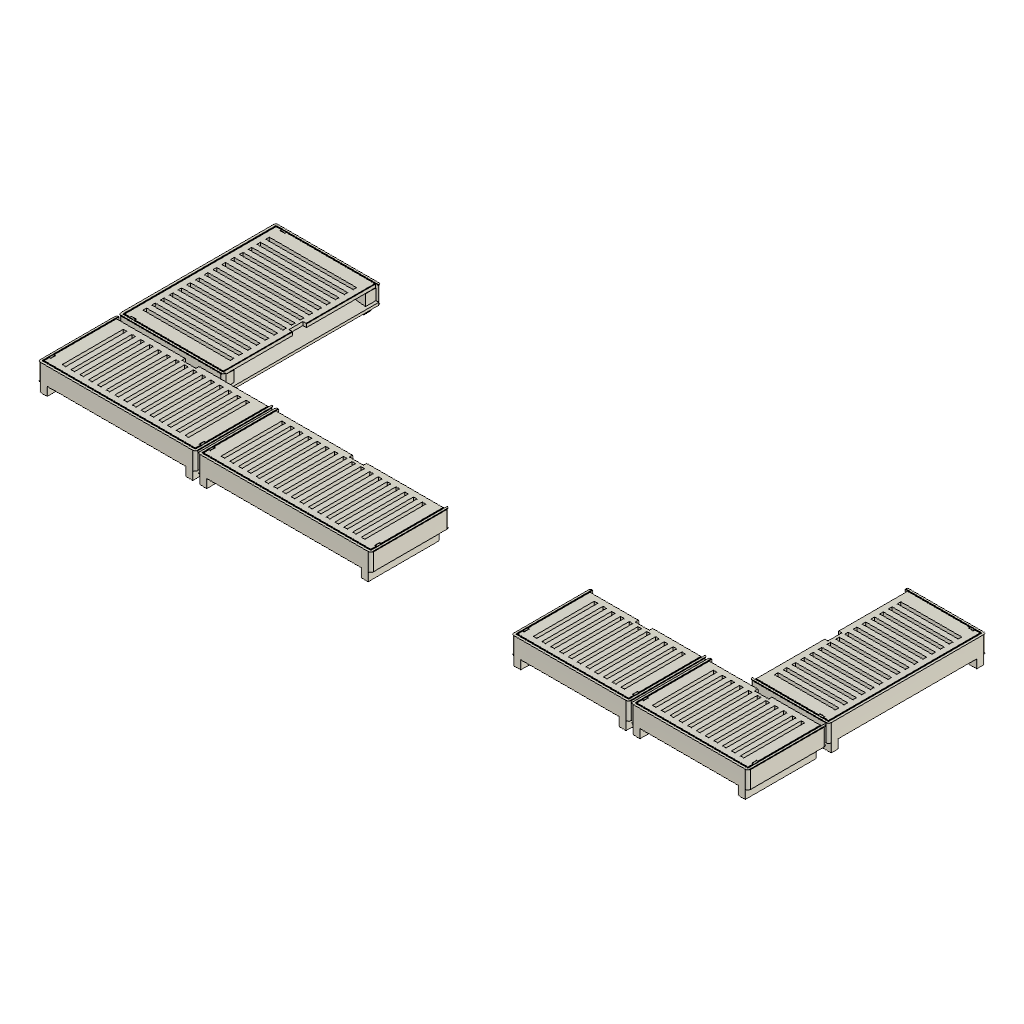
Sink_Organizer_B_R04_Single_Low (Autodesk Fusion 360 design; units mm, degrees)
Autodesk Fusion 360 part; units mm, degrees
(part 1 of 5)
ref_plane "工作平面1" through (0, 0, 10) normal (0, 0, 1) x (1, 0, 0) in component "R1_Integrated"
sketch "草图1" plane through (0, 0, 10) normal (0, 0, 1) x (1, 0, 0) in component "R1_Integrated"
  line L0 (590, 50) -> (724, 50)
  line L1 (724, 50) -> (724, 140)
  line L2 (724, 140) -> (590, 140)
  line L3 (590, 140) -> (590, 50)
  dimension "d43" = 590
  dimension "d44" = 50
  dimension "d45" = 134
  dimension "d46" = 90
  constraint horizontal L0
  constraint vertical L1
  constraint horizontal L2
  constraint vertical L3
  measures "d43" horizontal distance of origin L0.start
  measures "d44" vertical distance of origin L0.start
  measures "d45" horizontal distance of L0.start L0.end
  measures "d46" vertical distance of L0.end L1.end
extrude "R04 pan blank" add sketch "草图1" along normal blind 20 makes body 1 in component "R1_Integrated"
fillet "Outside corner rounds" radius 3 4 edges at (590, 140, 20) (724, 140, 20) (724, 50, 20) (590, 50, 20) on bodies 1 in component "R1_Integrated"
ref_plane "工作平面2" through (593, 0, 0) normal (1, 0, 0) x (0, 1, 0) in component "R1_Integrated"
sketch "草图2" plane through (593, 0, 0) normal (1, 0, 0) x (0, 0, -1) in component "R1_Integrated"
  line L0 (-22.1441, 53) -> (-13, 140)
  line L1 (-13, 140) -> (-31, 140)
  line L2 (-31, 140) -> (-31, 53)
  line L3 (-31, 53) -> (-22.1441, 53)
  dimension "d55" = 13
  dimension "d57" = 31
  constraint horizontal L1
  constraint vertical L2
  constraint horizontal L3
  measures "d55" horizontal distance of origin L0.end
  measures "d57" horizontal distance of origin L1.end
extrude "R04 continuous slope and open edge" cut sketch "草图2" along normal blind 128 bodies 1 in component "R1_Integrated"
ref_plane "工作平面3" through (0, 0, 10) normal (0, 0, 1) x (1, 0, 0) in component "R1_Integrated"
sketch "草图3" plane through (0, 0, 10) normal (0, 0, 1) x (1, 0, 0) in component "R1_Integrated"
  line L0 (593, 53) -> (605, 53)
  line L1 (605, 53) -> (605, 65)
  line L2 (605, 65) -> (593, 65)
  line L3 (593, 65) -> (593, 53)
  dimension "d64" = 12
  dimension "d65" = 12
  constraint horizontal L0
  constraint vertical L1
  constraint horizontal L2
  constraint vertical L3
  measures "d64" horizontal distance of L0.start L0.end
  measures "d65" vertical distance of L0.end L1.end
extrude "Grate seat 00" add sketch "草图3" along normal blind 16 bodies 1 in component "R1_Integrated"
ref_plane "工作平面4" through (0, 0, 10) normal (0, 0, 1) x (1, 0, 0) in component "R1_Integrated"
sketch "草图4" plane through (0, 0, 10) normal (0, 0, 1) x (1, 0, 0) in component "R1_Integrated"
  line L0 (593, 125) -> (605, 125)
  line L1 (605, 125) -> (605, 137)
  line L2 (605, 137) -> (593, 137)
  line L3 (593, 137) -> (593, 125)
  dimension "d71" = 125
  dimension "d72" = 12
  dimension "d73" = 12
  constraint horizontal L0
  constraint vertical L1
  constraint horizontal L2
  constraint vertical L3
  measures "d71" vertical distance of origin L0.start
  measures "d72" horizontal distance of L0.start L0.end
  measures "d73" vertical distance of L0.end L1.end
extrude "Grate seat 01" add sketch "草图4" along normal blind 16 bodies 1 in component "R1_Integrated"
ref_plane "工作平面5" through (0, 0, 10) normal (0, 0, 1) x (1, 0, 0) in component "R1_Integrated"
sketch "草图5" plane through (0, 0, 10) normal (0, 0, 1) x (1, 0, 0) in component "R1_Integrated"
  line L0 (709, 53) -> (721, 53)
  line L1 (721, 53) -> (721, 65)
  line L2 (721, 65) -> (709, 65)
  line L3 (709, 65) -> (709, 53)
  dimension "d78" = 709
  dimension "d80" = 12
  dimension "d81" = 12
  constraint horizontal L0
  constraint vertical L1
  constraint horizontal L2
  constraint vertical L3
  measures "d78" horizontal distance of origin L0.start
  measures "d80" horizontal distance of L0.start L0.end
  measures "d81" vertical distance of L0.end L1.end
extrude "Grate seat 10" add sketch "草图5" along normal blind 16 bodies 1 in component "R1_Integrated"
ref_plane "工作平面6" through (0, 0, 10) normal (0, 0, 1) x (1, 0, 0) in component "R1_Integrated"
sketch "草图6" plane through (0, 0, 10) normal (0, 0, 1) x (1, 0, 0) in component "R1_Integrated"
  line L0 (709, 125) -> (721, 125)
  line L1 (721, 125) -> (721, 137)
  line L2 (721, 137) -> (709, 137)
  line L3 (709, 137) -> (709, 125)
  dimension "d86" = 709
  dimension "d87" = 125
  dimension "d88" = 12
  dimension "d89" = 12
  constraint horizontal L0
  constraint vertical L1
  constraint horizontal L2
  constraint vertical L3
  measures "d86" horizontal distance of origin L0.start
  measures "d87" vertical distance of origin L0.start
  measures "d88" horizontal distance of L0.start L0.end
  measures "d89" vertical distance of L0.end L1.end
extrude "Grate seat 11" add sketch "草图6" along normal blind 16 bodies 1 in component "R1_Integrated"
ref_plane "工作平面7" through (0, 0, 0) normal (0, 0, 1) x (1, 0, 0) in component "R1_Integrated"
sketch "草图7" plane through (0, 0, 0) normal (0, 0, 1) x (1, 0, 0) in component "R1_Integrated"
  line L0 (593, 50) -> (601, 50)
  line L1 (601, 50) -> (601, 131)
  line L2 (601, 131) -> (593, 131)
  line L3 (593, 131) -> (593, 50)
  dimension "d94" = 593
  dimension "d95" = 50
  dimension "d96" = 8
  dimension "d97" = 81
  constraint horizontal L0
  constraint vertical L1
  constraint horizontal L2
  constraint vertical L3
  measures "d94" horizontal distance of origin L0.start
  measures "d95" vertical distance of origin L0.start
  measures "d96" horizontal distance of L0.start L0.end
  measures "d97" vertical distance of L0.end L1.end
extrude "R04 low integral runner 0" add sketch "草图7" along normal blind 10 bodies 1 in component "R1_Integrated"
ref_plane "工作平面8" through (0, 0, 0) normal (0, 0, 1) x (1, 0, 0) in component "R1_Integrated"
sketch "草图8" plane through (0, 0, 0) normal (0, 0, 1) x (1, 0, 0) in component "R1_Integrated"
  line L0 (713, 50) -> (721, 50)
  line L1 (721, 50) -> (721, 131)
  line L2 (721, 131) -> (713, 131)
  line L3 (713, 131) -> (713, 50)
  dimension "d102" = 713
  dimension "d103" = 50
  dimension "d104" = 8
  dimension "d105" = 81
  constraint horizontal L0
  constraint vertical L1
  constraint horizontal L2
  constraint vertical L3
  measures "d102" horizontal distance of origin L0.start
  measures "d103" vertical distance of origin L0.start
  measures "d104" horizontal distance of L0.start L0.end
  measures "d105" vertical distance of L0.end L1.end
extrude "R04 low integral runner 1" add sketch "草图8" along normal blind 10 bodies 1 in component "R1_Integrated"
chamfer "R03 touch edge chamfer" distance 0.4 angle 45 5 edges at (657, 53, 30) (593, 96.5, 30) (721, 96.5, 30) (590, 95, 30) (724, 95, 30) on bodies 1 in component "R1_Integrated"
ref_plane "工作平面1" through (0, 0, 26) normal (0, 0, 1) x (1, 0, 0) in component "R1_RemovableGrate"
sketch "草图1 (2)" plane through (0, 0, 26) normal (0, 0, 1) x (1, 0, 0) in component "R1_RemovableGrate"
  line L0 (593.3, 53.3) -> (720.7, 53.3)
  line L1 (720.7, 53.3) -> (720.7, 136.7)
  line L2 (720.7, 136.7) -> (593.3, 136.7)
  line L3 (593.3, 136.7) -> (593.3, 53.3)
  dimension "d113" = 127.4
  dimension "d114" = 83.4
  constraint horizontal L0
  constraint vertical L1
  constraint horizontal L2
  constraint vertical L3
  measures "d113" horizontal distance of L0.start L0.end
  measures "d114" vertical distance of L0.end L1.end
extrude "Horizontal removable deck" add sketch "草图1 (2)" along normal blind 4 separate body makes body 2 in component "R1_RemovableGrate"
ref_plane "工作平面2" through (0, 0, 26) normal (0, 0, 1) x (1, 0, 0) in component "R1_RemovableGrate"
sketch "草图2 (2)" plane through (0, 0, 26) normal (0, 0, 1) x (1, 0, 0) in component "R1_RemovableGrate"
  line L0 (605, 60.3) -> (609, 60.3)
  line L1 (609, 60.3) -> (609, 129.7)
  line L2 (609, 129.7) -> (605, 129.7)
  line L3 (605, 129.7) -> (605, 60.3)
  dimension "d119" = 605
  dimension "d121" = 4
  dimension "d122" = 69.4
  constraint horizontal L0
  constraint vertical L1
  constraint horizontal L2
  constraint vertical L3
  measures "d119" horizontal distance of origin L0.start
  measures "d121" horizontal distance of L0.start L0.end
  measures "d122" vertical distance of L0.end L1.end
extrude "Drain slot 1" cut sketch "草图2 (2)" along normal blind 4 bodies 2 in component "R1_RemovableGrate"
ref_plane "工作平面3" through (0, 0, 26) normal (0, 0, 1) x (1, 0, 0) in component "R1_RemovableGrate"
sketch "草图3 (2)" plane through (0, 0, 26) normal (0, 0, 1) x (1, 0, 0) in component "R1_RemovableGrate"
  line L0 (615, 60.3) -> (619, 60.3)
  line L1 (619, 60.3) -> (619, 129.7)
  line L2 (619, 129.7) -> (615, 129.7)
  line L3 (615, 129.7) -> (615, 60.3)
  dimension "d127" = 615
  dimension "d129" = 4
  dimension "d130" = 69.4
  constraint horizontal L0
  constraint vertical L1
  constraint horizontal L2
  constraint vertical L3
  measures "d127" horizontal distance of origin L0.start
  measures "d129" horizontal distance of L0.start L0.end
  measures "d130" vertical distance of L0.end L1.end
extrude "Drain slot 2" cut sketch "草图3 (2)" along normal blind 4 bodies 2 in component "R1_RemovableGrate"
ref_plane "工作平面4" through (0, 0, 26) normal (0, 0, 1) x (1, 0, 0) in component "R1_RemovableGrate"
sketch "草图4 (2)" plane through (0, 0, 26) normal (0, 0, 1) x (1, 0, 0) in component "R1_RemovableGrate"
  line L0 (625, 60.3) -> (629, 60.3)
  line L1 (629, 60.3) -> (629, 129.7)
  line L2 (629, 129.7) -> (625, 129.7)
  line L3 (625, 129.7) -> (625, 60.3)
  dimension "d135" = 625
  dimension "d137" = 4
  dimension "d138" = 69.4
  constraint horizontal L0
  constraint vertical L1
  constraint horizontal L2
  constraint vertical L3
  measures "d135" horizontal distance of origin L0.start
  measures "d137" horizontal distance of L0.start L0.end
  measures "d138" vertical distance of L0.end L1.end
extrude "Drain slot 3" cut sketch "草图4 (2)" along normal blind 4 bodies 2 in component "R1_RemovableGrate"
ref_plane "工作平面5" through (0, 0, 26) normal (0, 0, 1) x (1, 0, 0) in component "R1_RemovableGrate"
sketch "草图5 (2)" plane through (0, 0, 26) normal (0, 0, 1) x (1, 0, 0) in component "R1_RemovableGrate"
  line L0 (635, 60.3) -> (639, 60.3)
  line L1 (639, 60.3) -> (639, 129.7)
  line L2 (639, 129.7) -> (635, 129.7)
  line L3 (635, 129.7) -> (635, 60.3)
  dimension "d143" = 635
  dimension "d145" = 4
  dimension "d146" = 69.4
  constraint horizontal L0
  constraint vertical L1
  constraint horizontal L2
  constraint vertical L3
  measures "d143" horizontal distance of origin L0.start
  measures "d145" horizontal distance of L0.start L0.end
  measures "d146" vertical distance of L0.end L1.end
extrude "Drain slot 4" cut sketch "草图5 (2)" along normal blind 4 bodies 2 in component "R1_RemovableGrate"
ref_plane "工作平面6" through (0, 0, 26) normal (0, 0, 1) x (1, 0, 0) in component "R1_RemovableGrate"
sketch "草图6 (2)" plane through (0, 0, 26) normal (0, 0, 1) x (1, 0, 0) in component "R1_RemovableGrate"
  line L0 (645, 60.3) -> (649, 60.3)
  line L1 (649, 60.3) -> (649, 129.7)
  line L2 (649, 129.7) -> (645, 129.7)
  line L3 (645, 129.7) -> (645, 60.3)
  dimension "d151" = 645
  dimension "d153" = 4
  dimension "d154" = 69.4
  constraint horizontal L0
  constraint vertical L1
  constraint horizontal L2
  constraint vertical L3
  measures "d151" horizontal distance of origin L0.start
  measures "d153" horizontal distance of L0.start L0.end
  measures "d154" vertical distance of L0.end L1.end
extrude "Drain slot 5" cut sketch "草图6 (2)" along normal blind 4 bodies 2 in component "R1_RemovableGrate"
ref_plane "工作平面7" through (0, 0, 26) normal (0, 0, 1) x (1, 0, 0) in component "R1_RemovableGrate"
sketch "草图7 (2)" plane through (0, 0, 26) normal (0, 0, 1) x (1, 0, 0) in component "R1_RemovableGrate"
  line L0 (655, 60.3) -> (659, 60.3)
  line L1 (659, 60.3) -> (659, 129.7)
  line L2 (659, 129.7) -> (655, 129.7)
  line L3 (655, 129.7) -> (655, 60.3)
  dimension "d159" = 655
  dimension "d161" = 4
  dimension "d162" = 69.4
  constraint horizontal L0
  constraint vertical L1
  constraint horizontal L2
  constraint vertical L3
  measures "d159" horizontal distance of origin L0.start
  measures "d161" horizontal distance of L0.start L0.end
  measures "d162" vertical distance of L0.end L1.end
extrude "Drain slot 6" cut sketch "草图7 (2)" along normal blind 4 bodies 2 in component "R1_RemovableGrate"
ref_plane "工作平面8" through (0, 0, 26) normal (0, 0, 1) x (1, 0, 0) in component "R1_RemovableGrate"
sketch "草图8 (2)" plane through (0, 0, 26) normal (0, 0, 1) x (1, 0, 0) in component "R1_RemovableGrate"
  line L0 (665, 60.3) -> (669, 60.3)
  line L1 (669, 60.3) -> (669, 129.7)
  line L2 (669, 129.7) -> (665, 129.7)
  line L3 (665, 129.7) -> (665, 60.3)
  dimension "d167" = 665
  dimension "d169" = 4
  dimension "d170" = 69.4
  constraint horizontal L0
  constraint vertical L1
  constraint horizontal L2
  constraint vertical L3
  measures "d167" horizontal distance of origin L0.start
  measures "d169" horizontal distance of L0.start L0.end
  measures "d170" vertical distance of L0.end L1.end
extrude "Drain slot 7" cut sketch "草图8 (2)" along normal blind 4 bodies 2 in component "R1_RemovableGrate"
ref_plane "工作平面9" through (0, 0, 26) normal (0, 0, 1) x (1, 0, 0) in component "R1_RemovableGrate"
sketch "草图9" plane through (0, 0, 26) normal (0, 0, 1) x (1, 0, 0) in component "R1_RemovableGrate"
  line L0 (675, 60.3) -> (679, 60.3)
  line L1 (679, 60.3) -> (679, 129.7)
  line L2 (679, 129.7) -> (675, 129.7)
  line L3 (675, 129.7) -> (675, 60.3)
  dimension "d175" = 675
  dimension "d177" = 4
  dimension "d178" = 69.4
  constraint horizontal L0
  constraint vertical L1
  constraint horizontal L2
  constraint vertical L3
  measures "d175" horizontal distance of origin L0.start
  measures "d177" horizontal distance of L0.start L0.end
  measures "d178" vertical distance of L0.end L1.end
extrude "Drain slot 8" cut sketch "草图9" along normal blind 4 bodies 2 in component "R1_RemovableGrate"
ref_plane "工作平面10" through (0, 0, 26) normal (0, 0, 1) x (1, 0, 0) in component "R1_RemovableGrate"
sketch "草图10" plane through (0, 0, 26) normal (0, 0, 1) x (1, 0, 0) in component "R1_RemovableGrate"
  line L0 (685, 60.3) -> (689, 60.3)
  line L1 (689, 60.3) -> (689, 129.7)
  line L2 (689, 129.7) -> (685, 129.7)
  line L3 (685, 129.7) -> (685, 60.3)
  dimension "d183" = 685
  dimension "d185" = 4
  dimension "d186" = 69.4
  constraint horizontal L0
  constraint vertical L1
  constraint horizontal L2
  constraint vertical L3
  measures "d183" horizontal distance of origin L0.start
  measures "d185" horizontal distance of L0.start L0.end
  measures "d186" vertical distance of L0.end L1.end
extrude "Drain slot 9" cut sketch "草图10" along normal blind 4 bodies 2 in component "R1_RemovableGrate"
ref_plane "工作平面11" through (0, 0, 26) normal (0, 0, 1) x (1, 0, 0) in component "R1_RemovableGrate"
sketch "草图11" plane through (0, 0, 26) normal (0, 0, 1) x (1, 0, 0) in component "R1_RemovableGrate"
  line L0 (695, 60.3) -> (699, 60.3)
  line L1 (699, 60.3) -> (699, 129.7)
  line L2 (699, 129.7) -> (695, 129.7)
  line L3 (695, 129.7) -> (695, 60.3)
  dimension "d191" = 695
  dimension "d193" = 4
  dimension "d194" = 69.4
  constraint horizontal L0
  constraint vertical L1
  constraint horizontal L2
  constraint vertical L3
  measures "d191" horizontal distance of origin L0.start
  measures "d193" horizontal distance of L0.start L0.end
  measures "d194" vertical distance of L0.end L1.end
extrude "Drain slot 10" cut sketch "草图11" along normal blind 4 bodies 2 in component "R1_RemovableGrate"
ref_plane "工作平面12" through (0, 0, 26) normal (0, 0, 1) x (1, 0, 0) in component "R1_RemovableGrate"
sketch "草图12" plane through (0, 0, 26) normal (0, 0, 1) x (1, 0, 0) in component "R1_RemovableGrate"
  line L0 (705, 60.3) -> (709, 60.3)
  line L1 (709, 60.3) -> (709, 129.7)
  line L2 (709, 129.7) -> (705, 129.7)
  line L3 (705, 129.7) -> (705, 60.3)
  dimension "d199" = 705
  dimension "d201" = 4
  dimension "d202" = 69.4
  constraint horizontal L0
  constraint vertical L1
  constraint horizontal L2
  constraint vertical L3
  measures "d199" horizontal distance of origin L0.start
  measures "d201" horizontal distance of L0.start L0.end
  measures "d202" vertical distance of L0.end L1.end
extrude "Drain slot 11" cut sketch "草图12" along normal blind 4 bodies 2 in component "R1_RemovableGrate"
ref_plane "工作平面13" through (0, 0, 26) normal (0, 0, 1) x (1, 0, 0) in component "R1_RemovableGrate"
sketch "草图13" plane through (0, 0, 26) normal (0, 0, 1) x (1, 0, 0) in component "R1_RemovableGrate"
  line L0 (649, 132.7) -> (665, 132.7)
  line L1 (665, 132.7) -> (665, 137.7)
  line L2 (665, 137.7) -> (649, 137.7)
  line L3 (649, 137.7) -> (649, 132.7)
  dimension "d207" = 649
  dimension "d208" = 132.7
  dimension "d209" = 16
  dimension "d210" = 5
  constraint horizontal L0
  constraint vertical L1
  constraint horizontal L2
  constraint vertical L3
  measures "d207" horizontal distance of origin L0.start
  measures "d208" vertical distance of origin L0.start
  measures "d209" horizontal distance of L0.start L0.end
  measures "d210" vertical distance of L0.end L1.end
extrude "Finger lift notch" cut sketch "草图13" along normal blind 4 bodies 2 in component "R1_RemovableGrate"
chamfer "R03 touch edge chamfer'" distance 0.4 angle 45 5 edges at (621.15, 136.7, 30) (593.3, 95, 30) (657, 53.3, 30) (720.7, 95, 30) (692.85, 136.7, 30) on bodies 2 in component "R1_RemovableGrate"
ref_plane "工作平面1" through (0, 0, 10) normal (0, 0, 1) x (1, 0, 0) in component "L1_Integrated"
sketch "草图1 (3)" plane through (0, 0, 10) normal (0, 0, 1) x (1, 0, 0) in component "L1_Integrated"
  line L0 (50, 50) -> (230, 50)
  line L1 (230, 50) -> (230, 140)
  line L2 (230, 140) -> (50, 140)
  line L3 (50, 140) -> (50, 50)
  dimension "d216" = 50
  dimension "d217" = 50
  dimension "d218" = 180
  dimension "d219" = 90
  constraint horizontal L0
  constraint vertical L1
  constraint horizontal L2
  constraint vertical L3
  measures "d216" horizontal distance of origin L0.start
  measures "d217" vertical distance of origin L0.start
  measures "d218" horizontal distance of L0.start L0.end
  measures "d219" vertical distance of L0.end L1.end
extrude "R04 pan blank'" add sketch "草图1 (3)" along normal blind 20 separate body makes body 3 in component "L1_Integrated"
fillet "Outside corner rounds'" radius 3 4 edges at (50, 140, 20) (230, 140, 20) (230, 50, 20) (50, 50, 20) on bodies 3 in component "L1_Integrated"
ref_plane "工作平面2" through (53, 0, 0) normal (1, 0, 0) x (0, 1, 0) in component "L1_Integrated"
sketch "草图2 (3)" plane through (53, 0, 0) normal (1, 0, 0) x (0, 0, -1) in component "L1_Integrated"
  line L0 (-22.1441, 53) -> (-13, 140)
  line L1 (-13, 140) -> (-31, 140)
  line L2 (-31, 140) -> (-31, 53)
  line L3 (-31, 53) -> (-22.1441, 53)
  dimension "d228" = 13
  dimension "d230" = 31
  constraint horizontal L1
  constraint vertical L2
  constraint horizontal L3
  measures "d228" horizontal distance of origin L0.end
  measures "d230" horizontal distance of origin L1.end
extrude "R04 continuous slope and open edge'" cut sketch "草图2 (3)" along normal blind 174 bodies 3 in component "L1_Integrated"
ref_plane "工作平面3" through (0, 0, 10) normal (0, 0, 1) x (1, 0, 0) in component "L1_Integrated"
sketch "草图3 (3)" plane through (0, 0, 10) normal (0, 0, 1) x (1, 0, 0) in component "L1_Integrated"
  line L0 (53, 53) -> (65, 53)
  line L1 (65, 53) -> (65, 65)
  line L2 (65, 65) -> (53, 65)
  line L3 (53, 65) -> (53, 53)
  dimension "d237" = 12
  dimension "d238" = 12
  constraint horizontal L0
  constraint vertical L1
  constraint horizontal L2
  constraint vertical L3
  measures "d237" horizontal distance of L0.start L0.end
  measures "d238" vertical distance of L0.end L1.end
extrude "Grate seat 00'" add sketch "草图3 (3)" along normal blind 16 bodies 3 in component "L1_Integrated"
ref_plane "工作平面4" through (0, 0, 10) normal (0, 0, 1) x (1, 0, 0) in component "L1_Integrated"
sketch "草图4 (3)" plane through (0, 0, 10) normal (0, 0, 1) x (1, 0, 0) in component "L1_Integrated"
  line L0 (53, 125) -> (65, 125)
  line L1 (65, 125) -> (65, 137)
  line L2 (65, 137) -> (53, 137)
  line L3 (53, 137) -> (53, 125)
  dimension "d244" = 125
  dimension "d245" = 12
  dimension "d246" = 12
  constraint horizontal L0
  constraint vertical L1
  constraint horizontal L2
  constraint vertical L3
  measures "d244" vertical distance of origin L0.start
  measures "d245" horizontal distance of L0.start L0.end
  measures "d246" vertical distance of L0.end L1.end
extrude "Grate seat 01'" add sketch "草图4 (3)" along normal blind 16 bodies 3 in component "L1_Integrated"
ref_plane "工作平面5" through (0, 0, 10) normal (0, 0, 1) x (1, 0, 0) in component "L1_Integrated"
sketch "草图5 (3)" plane through (0, 0, 10) normal (0, 0, 1) x (1, 0, 0) in component "L1_Integrated"
  line L0 (215, 53) -> (227, 53)
  line L1 (227, 53) -> (227, 65)
  line L2 (227, 65) -> (215, 65)
  line L3 (215, 65) -> (215, 53)
  dimension "d251" = 215
  dimension "d253" = 12
  dimension "d254" = 12
  constraint horizontal L0
  constraint vertical L1
  constraint horizontal L2
  constraint vertical L3
  measures "d251" horizontal distance of origin L0.start
  measures "d253" horizontal distance of L0.start L0.end
  measures "d254" vertical distance of L0.end L1.end
extrude "Grate seat 10'" add sketch "草图5 (3)" along normal blind 16 bodies 3 in component "L1_Integrated"
ref_plane "工作平面6" through (0, 0, 10) normal (0, 0, 1) x (1, 0, 0) in component "L1_Integrated"
sketch "草图6 (3)" plane through (0, 0, 10) normal (0, 0, 1) x (1, 0, 0) in component "L1_Integrated"
  line L0 (215, 125) -> (227, 125)
  line L1 (227, 125) -> (227, 137)
  line L2 (227, 137) -> (215, 137)
  line L3 (215, 137) -> (215, 125)
  dimension "d259" = 215
  dimension "d260" = 125
  dimension "d261" = 12
  dimension "d262" = 12
  constraint horizontal L0
  constraint vertical L1
  constraint horizontal L2
  constraint vertical L3
  measures "d259" horizontal distance of origin L0.start
  measures "d260" vertical distance of origin L0.start
  measures "d261" horizontal distance of L0.start L0.end
  measures "d262" vertical distance of L0.end L1.end
extrude "Grate seat 11'" add sketch "草图6 (3)" along normal blind 16 bodies 3 in component "L1_Integrated"
ref_plane "工作平面7" through (0, 0, 0) normal (0, 0, 1) x (1, 0, 0) in component "L1_Integrated"
sketch "草图7 (3)" plane through (0, 0, 0) normal (0, 0, 1) x (1, 0, 0) in component "L1_Integrated"
  line L0 (53, 50) -> (61, 50)
  line L1 (61, 50) -> (61, 131)
  line L2 (61, 131) -> (53, 131)
  line L3 (53, 131) -> (53, 50)
  dimension "d267" = 53
  dimension "d268" = 50
  dimension "d269" = 8
  dimension "d270" = 81
  constraint horizontal L0
  constraint vertical L1
  constraint horizontal L2
  constraint vertical L3
  measures "d267" horizontal distance of origin L0.start
  measures "d268" vertical distance of origin L0.start
  measures "d269" horizontal distance of L0.start L0.end
  measures "d270" vertical distance of L0.end L1.end
extrude "R04 low integral runner 0'" add sketch "草图7 (3)" along normal blind 10 bodies 3 in component "L1_Integrated"
ref_plane "工作平面8" through (0, 0, 0) normal (0, 0, 1) x (1, 0, 0) in component "L1_Integrated"
sketch "草图8 (3)" plane through (0, 0, 0) normal (0, 0, 1) x (1, 0, 0) in component "L1_Integrated"
  line L0 (219, 50) -> (227, 50)
  line L1 (227, 50) -> (227, 131)
  line L2 (227, 131) -> (219, 131)
  line L3 (219, 131) -> (219, 50)
  dimension "d275" = 219
  dimension "d276" = 50
  dimension "d277" = 8
  dimension "d278" = 81
  constraint horizontal L0
  constraint vertical L1
  constraint horizontal L2
  constraint vertical L3
  measures "d275" horizontal distance of origin L0.start
  measures "d276" vertical distance of origin L0.start
  measures "d277" horizontal distance of L0.start L0.end
  measures "d278" vertical distance of L0.end L1.end
extrude "R04 low integral runner 1'" add sketch "草图8 (3)" along normal blind 10 bodies 3 in component "L1_Integrated"
chamfer "R03 touch edge chamfer''" distance 0.4 angle 45 5 edges at (140, 53, 30) (53, 96.5, 30) (227, 96.5, 30) (50, 95, 30) (230, 95, 30) on bodies 3 in component "L1_Integrated"
ref_plane "工作平面1" through (0, 0, 26) normal (0, 0, 1) x (1, 0, 0) in component "L1_RemovableGrate"
sketch "草图1 (4)" plane through (0, 0, 26) normal (0, 0, 1) x (1, 0, 0) in component "L1_RemovableGrate"
  line L0 (53.3, 53.3) -> (226.7, 53.3)
  line L1 (226.7, 53.3) -> (226.7, 136.7)
  line L2 (226.7, 136.7) -> (53.3, 136.7)
  line L3 (53.3, 136.7) -> (53.3, 53.3)
  dimension "d286" = 173.4
  dimension "d287" = 83.4
  constraint horizontal L0
  constraint vertical L1
  constraint horizontal L2
  constraint vertical L3
  measures "d286" horizontal distance of L0.start L0.end
  measures "d287" vertical distance of L0.end L1.end
extrude "Horizontal removable deck'" add sketch "草图1 (4)" along normal blind 4 separate body makes body 4 in component "L1_RemovableGrate"
ref_plane "工作平面2" through (0, 0, 26) normal (0, 0, 1) x (1, 0, 0) in component "L1_RemovableGrate"
sketch "草图2 (4)" plane through (0, 0, 26) normal (0, 0, 1) x (1, 0, 0) in component "L1_RemovableGrate"
  line L0 (68, 60.3) -> (72, 60.3)
  line L1 (72, 60.3) -> (72, 129.7)
  line L2 (72, 129.7) -> (68, 129.7)
  line L3 (68, 129.7) -> (68, 60.3)
  dimension "d292" = 68
  dimension "d294" = 4
  dimension "d295" = 69.4
  constraint horizontal L0
  constraint vertical L1
  constraint horizontal L2
  constraint vertical L3
  measures "d292" horizontal distance of origin L0.start
  measures "d294" horizontal distance of L0.start L0.end
  measures "d295" vertical distance of L0.end L1.end
extrude "Drain slot 1'" cut sketch "草图2 (4)" along normal blind 4 bodies 4 in component "L1_RemovableGrate"
ref_plane "工作平面3" through (0, 0, 26) normal (0, 0, 1) x (1, 0, 0) in component "L1_RemovableGrate"
sketch "草图3 (4)" plane through (0, 0, 26) normal (0, 0, 1) x (1, 0, 0) in component "L1_RemovableGrate"
  line L0 (78, 60.3) -> (82, 60.3)
  line L1 (82, 60.3) -> (82, 129.7)
  line L2 (82, 129.7) -> (78, 129.7)
  line L3 (78, 129.7) -> (78, 60.3)
  dimension "d300" = 78
  dimension "d302" = 4
  dimension "d303" = 69.4
  constraint horizontal L0
  constraint vertical L1
  constraint horizontal L2
  constraint vertical L3
  measures "d300" horizontal distance of origin L0.start
  measures "d302" horizontal distance of L0.start L0.end
  measures "d303" vertical distance of L0.end L1.end
extrude "Drain slot 2'" cut sketch "草图3 (4)" along normal blind 4 bodies 4 in component "L1_RemovableGrate"
ref_plane "工作平面4" through (0, 0, 26) normal (0, 0, 1) x (1, 0, 0) in component "L1_RemovableGrate"
sketch "草图4 (4)" plane through (0, 0, 26) normal (0, 0, 1) x (1, 0, 0) in component "L1_RemovableGrate"
  line L0 (88, 60.3) -> (92, 60.3)
  line L1 (92, 60.3) -> (92, 129.7)
  line L2 (92, 129.7) -> (88, 129.7)
  line L3 (88, 129.7) -> (88, 60.3)
  dimension "d308" = 88
  dimension "d310" = 4
  dimension "d311" = 69.4
  constraint horizontal L0
  constraint vertical L1
  constraint horizontal L2
  constraint vertical L3
  measures "d308" horizontal distance of origin L0.start
  measures "d310" horizontal distance of L0.start L0.end
  measures "d311" vertical distance of L0.end L1.end
extrude "Drain slot 3'" cut sketch "草图4 (4)" along normal blind 4 bodies 4 in component "L1_RemovableGrate"
ref_plane "工作平面5" through (0, 0, 26) normal (0, 0, 1) x (1, 0, 0) in component "L1_RemovableGrate"
sketch "草图5 (4)" plane through (0, 0, 26) normal (0, 0, 1) x (1, 0, 0) in component "L1_RemovableGrate"
  line L0 (98, 60.3) -> (102, 60.3)
  line L1 (102, 60.3) -> (102, 129.7)
  line L2 (102, 129.7) -> (98, 129.7)
  line L3 (98, 129.7) -> (98, 60.3)
  dimension "d316" = 98
  dimension "d318" = 4
  dimension "d319" = 69.4
  constraint horizontal L0
  constraint vertical L1
  constraint horizontal L2
  constraint vertical L3
  measures "d316" horizontal distance of origin L0.start
  measures "d318" horizontal distance of L0.start L0.end
  measures "d319" vertical distance of L0.end L1.end
extrude "Drain slot 4'" cut sketch "草图5 (4)" along normal blind 4 bodies 4 in component "L1_RemovableGrate"
ref_plane "工作平面6" through (0, 0, 26) normal (0, 0, 1) x (1, 0, 0) in component "L1_RemovableGrate"
sketch "草图6 (4)" plane through (0, 0, 26) normal (0, 0, 1) x (1, 0, 0) in component "L1_RemovableGrate"
  line L0 (108, 60.3) -> (112, 60.3)
  line L1 (112, 60.3) -> (112, 129.7)
  line L2 (112, 129.7) -> (108, 129.7)
  line L3 (108, 129.7) -> (108, 60.3)
  dimension "d324" = 108
  dimension "d326" = 4
  dimension "d327" = 69.4
  constraint horizontal L0
  constraint vertical L1
  constraint horizontal L2
  constraint vertical L3
  measures "d324" horizontal distance of origin L0.start
  measures "d326" horizontal distance of L0.start L0.end
  measures "d327" vertical distance of L0.end L1.end
extrude "Drain slot 5'" cut sketch "草图6 (4)" along normal blind 4 bodies 4 in component "L1_RemovableGrate"
ref_plane "工作平面7" through (0, 0, 26) normal (0, 0, 1) x (1, 0, 0) in component "L1_RemovableGrate"
sketch "草图7 (4)" plane through (0, 0, 26) normal (0, 0, 1) x (1, 0, 0) in component "L1_RemovableGrate"
  line L0 (118, 60.3) -> (122, 60.3)
  line L1 (122, 60.3) -> (122, 129.7)
  line L2 (122, 129.7) -> (118, 129.7)
  line L3 (118, 129.7) -> (118, 60.3)
  dimension "d332" = 118
  dimension "d334" = 4
  dimension "d335" = 69.4
  constraint horizontal L0
  constraint vertical L1
  constraint horizontal L2
  constraint vertical L3
  measures "d332" horizontal distance of origin L0.start
  measures "d334" horizontal distance of L0.start L0.end
  measures "d335" vertical distance of L0.end L1.end
extrude "Drain slot 6'" cut sketch "草图7 (4)" along normal blind 4 bodies 4 in component "L1_RemovableGrate"
ref_plane "工作平面8" through (0, 0, 26) normal (0, 0, 1) x (1, 0, 0) in component "L1_RemovableGrate"
sketch "草图8 (4)" plane through (0, 0, 26) normal (0, 0, 1) x (1, 0, 0) in component "L1_RemovableGrate"
  line L0 (128, 60.3) -> (132, 60.3)
  line L1 (132, 60.3) -> (132, 129.7)
  line L2 (132, 129.7) -> (128, 129.7)
  line L3 (128, 129.7) -> (128, 60.3)
  dimension "d340" = 128
  dimension "d342" = 4
  dimension "d343" = 69.4
  constraint horizontal L0
  constraint vertical L1
  constraint horizontal L2
  constraint vertical L3
  measures "d340" horizontal distance of origin L0.start
  measures "d342" horizontal distance of L0.start L0.end
  measures "d343" vertical distance of L0.end L1.end
extrude "Drain slot 7'" cut sketch "草图8 (4)" along normal blind 4 bodies 4 in component "L1_RemovableGrate"
ref_plane "工作平面9" through (0, 0, 26) normal (0, 0, 1) x (1, 0, 0) in component "L1_RemovableGrate"
sketch "草图9 (2)" plane through (0, 0, 26) normal (0, 0, 1) x (1, 0, 0) in component "L1_RemovableGrate"
  line L0 (138, 60.3) -> (142, 60.3)
  line L1 (142, 60.3) -> (142, 129.7)
  line L2 (142, 129.7) -> (138, 129.7)
  line L3 (138, 129.7) -> (138, 60.3)
  dimension "d348" = 138
  dimension "d350" = 4
  dimension "d351" = 69.4
  constraint horizontal L0
  constraint vertical L1
  constraint horizontal L2
  constraint vertical L3
  measures "d348" horizontal distance of origin L0.start
  measures "d350" horizontal distance of L0.start L0.end
  measures "d351" vertical distance of L0.end L1.end
extrude "Drain slot 8'" cut sketch "草图9 (2)" along normal blind 4 bodies 4 in component "L1_RemovableGrate"
ref_plane "工作平面10" through (0, 0, 26) normal (0, 0, 1) x (1, 0, 0) in component "L1_RemovableGrate"
sketch "草图10 (2)" plane through (0, 0, 26) normal (0, 0, 1) x (1, 0, 0) in component "L1_RemovableGrate"
  line L0 (148, 60.3) -> (152, 60.3)
  line L1 (152, 60.3) -> (152, 129.7)
  line L2 (152, 129.7) -> (148, 129.7)
  line L3 (148, 129.7) -> (148, 60.3)
  dimension "d356" = 148
  dimension "d358" = 4
  dimension "d359" = 69.4
  constraint horizontal L0
  constraint vertical L1
  constraint horizontal L2
  constraint vertical L3
  measures "d356" horizontal distance of origin L0.start
  measures "d358" horizontal distance of L0.start L0.end
  measures "d359" vertical distance of L0.end L1.end
extrude "Drain slot 9'" cut sketch "草图10 (2)" along normal blind 4 bodies 4 in component "L1_RemovableGrate"
ref_plane "工作平面11" through (0, 0, 26) normal (0, 0, 1) x (1, 0, 0) in component "L1_RemovableGrate"
sketch "草图11 (2)" plane through (0, 0, 26) normal (0, 0, 1) x (1, 0, 0) in component "L1_RemovableGrate"
  line L0 (158, 60.3) -> (162, 60.3)
  line L1 (162, 60.3) -> (162, 129.7)
  line L2 (162, 129.7) -> (158, 129.7)
  line L3 (158, 129.7) -> (158, 60.3)
  dimension "d364" = 158
  dimension "d366" = 4
  dimension "d367" = 69.4
  constraint horizontal L0
  constraint vertical L1
  constraint horizontal L2
  constraint vertical L3
  measures "d364" horizontal distance of origin L0.start
  measures "d366" horizontal distance of L0.start L0.end
  measures "d367" vertical distance of L0.end L1.end
extrude "Drain slot 10'" cut sketch "草图11 (2)" along normal blind 4 bodies 4 in component "L1_RemovableGrate"
ref_plane "工作平面12" through (0, 0, 26) normal (0, 0, 1) x (1, 0, 0) in component "L1_RemovableGrate"
sketch "草图12 (2)" plane through (0, 0, 26) normal (0, 0, 1) x (1, 0, 0) in component "L1_RemovableGrate"
  line L0 (168, 60.3) -> (172, 60.3)
  line L1 (172, 60.3) -> (172, 129.7)
  line L2 (172, 129.7) -> (168, 129.7)
  line L3 (168, 129.7) -> (168, 60.3)
  dimension "d372" = 168
  dimension "d374" = 4
  dimension "d375" = 69.4
  constraint horizontal L0
  constraint vertical L1
  constraint horizontal L2
  constraint vertical L3
  measures "d372" horizontal distance of origin L0.start
  measures "d374" horizontal distance of L0.start L0.end
  measures "d375" vertical distance of L0.end L1.end
extrude "Drain slot 11'" cut sketch "草图12 (2)" along normal blind 4 bodies 4 in component "L1_RemovableGrate"
ref_plane "工作平面13" through (0, 0, 26) normal (0, 0, 1) x (1, 0, 0) in component "L1_RemovableGrate"
sketch "草图13 (2)" plane through (0, 0, 26) normal (0, 0, 1) x (1, 0, 0) in component "L1_RemovableGrate"
  line L0 (178, 60.3) -> (182, 60.3)
  line L1 (182, 60.3) -> (182, 129.7)
  line L2 (182, 129.7) -> (178, 129.7)
  line L3 (178, 129.7) -> (178, 60.3)
  dimension "d380" = 178
  dimension "d382" = 4
  dimension "d383" = 69.4
  constraint horizontal L0
  constraint vertical L1
  constraint horizontal L2
  constraint vertical L3
  measures "d380" horizontal distance of origin L0.start
  measures "d382" horizontal distance of L0.start L0.end
  measures "d383" vertical distance of L0.end L1.end
extrude "Drain slot 12" cut sketch "草图13 (2)" along normal blind 4 bodies 4 in component "L1_RemovableGrate"
ref_plane "工作平面14" through (0, 0, 26) normal (0, 0, 1) x (1, 0, 0) in component "L1_RemovableGrate"
sketch "草图14" plane through (0, 0, 26) normal (0, 0, 1) x (1, 0, 0) in component "L1_RemovableGrate"
  line L0 (188, 60.3) -> (192, 60.3)
  line L1 (192, 60.3) -> (192, 129.7)
  line L2 (192, 129.7) -> (188, 129.7)
  line L3 (188, 129.7) -> (188, 60.3)
  dimension "d388" = 188
  dimension "d390" = 4
  dimension "d391" = 69.4
  constraint horizontal L0
  constraint vertical L1
  constraint horizontal L2
  constraint vertical L3
  measures "d388" horizontal distance of origin L0.start
  measures "d390" horizontal distance of L0.start L0.end
  measures "d391" vertical distance of L0.end L1.end
extrude "Drain slot 13" cut sketch "草图14" along normal blind 4 bodies 4 in component "L1_RemovableGrate"
ref_plane "工作平面15" through (0, 0, 26) normal (0, 0, 1) x (1, 0, 0) in component "L1_RemovableGrate"
sketch "草图15" plane through (0, 0, 26) normal (0, 0, 1) x (1, 0, 0) in component "L1_RemovableGrate"
  line L0 (198, 60.3) -> (202, 60.3)
  line L1 (202, 60.3) -> (202, 129.7)
  line L2 (202, 129.7) -> (198, 129.7)
  line L3 (198, 129.7) -> (198, 60.3)
  dimension "d396" = 198
  dimension "d398" = 4
  dimension "d399" = 69.4
  constraint horizontal L0
  constraint vertical L1
  constraint horizontal L2
  constraint vertical L3
  measures "d396" horizontal distance of origin L0.start
  measures "d398" horizontal distance of L0.start L0.end
  measures "d399" vertical distance of L0.end L1.end
extrude "Drain slot 14" cut sketch "草图15" along normal blind 4 bodies 4 in component "L1_RemovableGrate"
ref_plane "工作平面16" through (0, 0, 26) normal (0, 0, 1) x (1, 0, 0) in component "L1_RemovableGrate"
sketch "草图16" plane through (0, 0, 26) normal (0, 0, 1) x (1, 0, 0) in component "L1_RemovableGrate"
  line L0 (208, 60.3) -> (212, 60.3)
  line L1 (212, 60.3) -> (212, 129.7)
  line L2 (212, 129.7) -> (208, 129.7)
  line L3 (208, 129.7) -> (208, 60.3)
  dimension "d404" = 208
  dimension "d406" = 4
  dimension "d407" = 69.4
  constraint horizontal L0
  constraint vertical L1
  constraint horizontal L2
  constraint vertical L3
  measures "d404" horizontal distance of origin L0.start
  measures "d406" horizontal distance of L0.start L0.end
  measures "d407" vertical distance of L0.end L1.end
extrude "Drain slot 15" cut sketch "草图16" along normal blind 4 bodies 4 in component "L1_RemovableGrate"
ref_plane "工作平面17" through (0, 0, 26) normal (0, 0, 1) x (1, 0, 0) in component "L1_RemovableGrate"
sketch "草图17" plane through (0, 0, 26) normal (0, 0, 1) x (1, 0, 0) in component "L1_RemovableGrate"
  line L0 (132, 132.7) -> (148, 132.7)
  line L1 (148, 132.7) -> (148, 137.7)
  line L2 (148, 137.7) -> (132, 137.7)
  line L3 (132, 137.7) -> (132, 132.7)
  dimension "d412" = 132
  dimension "d413" = 132.7
  dimension "d414" = 16
  dimension "d415" = 5
  constraint horizontal L0
  constraint vertical L1
  constraint horizontal L2
  constraint vertical L3
  measures "d412" horizontal distance of origin L0.start
  measures "d413" vertical distance of origin L0.start
  measures "d414" horizontal distance of L0.start L0.end
  measures "d415" vertical distance of L0.end L1.end
extrude "Finger lift notch'" cut sketch "草图17" along normal blind 4 bodies 4 in component "L1_RemovableGrate"
chamfer "R03 touch edge chamfer'''" distance 0.4 angle 45 5 edges at (92.65, 136.7, 30) (53.3, 95, 30) (140, 53.3, 30) (226.7, 95, 30) (187.35, 136.7, 30) on bodies 4 in component "L1_RemovableGrate"
ref_plane "工作平面1" through (0, 0, 10) normal (0, 0, 1) x (1, 0, 0) in component "L2_Integrated"
sketch "草图1 (5)" plane through (0, 0, 10) normal (0, 0, 1) x (1, 0, 0) in component "L2_Integrated"
  line L0 (232, 50) -> (430, 50)
  line L1 (430, 50) -> (430, 140)
  line L2 (430, 140) -> (232, 140)
  line L3 (232, 140) -> (232, 50)
  dimension "d421" = 232
  dimension "d422" = 50
  dimension "d423" = 198
  dimension "d424" = 90
  constraint horizontal L0
  constraint vertical L1
  constraint horizontal L2
  constraint vertical L3
  measures "d421" horizontal distance of origin L0.start
  measures "d422" vertical distance of origin L0.start
  measures "d423" horizontal distance of L0.start L0.end
  measures "d424" vertical distance of L0.end L1.end
extrude "R04 pan blank''" add sketch "草图1 (5)" along normal blind 20 separate body makes body 5 in component "L2_Integrated"
fillet "Outside corner rounds''" radius 3 4 edges at (232, 140, 20) (430, 140, 20) (430, 50, 20) (232, 50, 20) on bodies 5 in component "L2_Integrated"
ref_plane "工作平面2" through (235, 0, 0) normal (1, 0, 0) x (0, 1, 0) in component "L2_Integrated"
sketch "草图2 (5)" plane through (235, 0, 0) normal (1, 0, 0) x (0, 0, -1) in component "L2_Integrated"
  line L0 (-22.1441, 53) -> (-13, 140)
  line L1 (-13, 140) -> (-31, 140)
  line L2 (-31, 140) -> (-31, 53)
  line L3 (-31, 53) -> (-22.1441, 53)
  dimension "d433" = 13
  dimension "d435" = 31
  constraint horizontal L1
  constraint vertical L2
  constraint horizontal L3
  measures "d433" horizontal distance of origin L0.end
  measures "d435" horizontal distance of origin L1.end
extrude "R04 continuous slope and open edge''" cut sketch "草图2 (5)" along normal blind 192 bodies 5 in component "L2_Integrated"
ref_plane "工作平面3" through (0, 0, 10) normal (0, 0, 1) x (1, 0, 0) in component "L2_Integrated"
sketch "草图3 (5)" plane through (0, 0, 10) normal (0, 0, 1) x (1, 0, 0) in component "L2_Integrated"
  line L0 (235, 53) -> (247, 53)
  line L1 (247, 53) -> (247, 65)
  line L2 (247, 65) -> (235, 65)
  line L3 (235, 65) -> (235, 53)
  dimension "d442" = 12
  dimension "d443" = 12
  constraint horizontal L0
  constraint vertical L1
  constraint horizontal L2
  constraint vertical L3
  measures "d442" horizontal distance of L0.start L0.end
  measures "d443" vertical distance of L0.end L1.end
extrude "Grate seat 00''" add sketch "草图3 (5)" along normal blind 16 bodies 5 in component "L2_Integrated"
ref_plane "工作平面4" through (0, 0, 10) normal (0, 0, 1) x (1, 0, 0) in component "L2_Integrated"
sketch "草图4 (5)" plane through (0, 0, 10) normal (0, 0, 1) x (1, 0, 0) in component "L2_Integrated"
  line L0 (235, 125) -> (247, 125)
  line L1 (247, 125) -> (247, 137)
  line L2 (247, 137) -> (235, 137)
  line L3 (235, 137) -> (235, 125)
  dimension "d449" = 125
  dimension "d450" = 12
  dimension "d451" = 12
  constraint horizontal L0
  constraint vertical L1
  constraint horizontal L2
  constraint vertical L3
  measures "d449" vertical distance of origin L0.start
  measures "d450" horizontal distance of L0.start L0.end
  measures "d451" vertical distance of L0.end L1.end
extrude "Grate seat 01''" add sketch "草图4 (5)" along normal blind 16 bodies 5 in component "L2_Integrated"
ref_plane "工作平面5" through (0, 0, 10) normal (0, 0, 1) x (1, 0, 0) in component "L2_Integrated"
sketch "草图5 (5)" plane through (0, 0, 10) normal (0, 0, 1) x (1, 0, 0) in component "L2_Integrated"
  line L0 (415, 53) -> (427, 53)
  line L1 (427, 53) -> (427, 65)
  line L2 (427, 65) -> (415, 65)
  line L3 (415, 65) -> (415, 53)
  dimension "d456" = 415
  dimension "d458" = 12
  dimension "d459" = 12
  constraint horizontal L0
  constraint vertical L1
  constraint horizontal L2
  constraint vertical L3
  measures "d456" horizontal distance of origin L0.start
  measures "d458" horizontal distance of L0.start L0.end
  measures "d459" vertical distance of L0.end L1.end
extrude "Grate seat 10''" add sketch "草图5 (5)" along normal blind 16 bodies 5 in component "L2_Integrated"
ref_plane "工作平面6" through (0, 0, 10) normal (0, 0, 1) x (1, 0, 0) in component "L2_Integrated"
sketch "草图6 (5)" plane through (0, 0, 10) normal (0, 0, 1) x (1, 0, 0) in component "L2_Integrated"
  line L0 (415, 125) -> (427, 125)
  line L1 (427, 125) -> (427, 137)
  line L2 (427, 137) -> (415, 137)
  line L3 (415, 137) -> (415, 125)
  dimension "d464" = 415
  dimension "d465" = 125
  dimension "d466" = 12
  dimension "d467" = 12
  constraint horizontal L0
  constraint vertical L1
  constraint horizontal L2
  constraint vertical L3
  measures "d464" horizontal distance of origin L0.start
  measures "d465" vertical distance of origin L0.start
  measures "d466" horizontal distance of L0.start L0.end
  measures "d467" vertical distance of L0.end L1.end
extrude "Grate seat 11''" add sketch "草图6 (5)" along normal blind 16 bodies 5 in component "L2_Integrated"
ref_plane "工作平面7" through (0, 0, 0) normal (0, 0, 1) x (1, 0, 0) in component "L2_Integrated"
sketch "草图7 (5)" plane through (0, 0, 0) normal (0, 0, 1) x (1, 0, 0) in component "L2_Integrated"
  line L0 (235, 50) -> (243, 50)
  line L1 (243, 50) -> (243, 131)
  line L2 (243, 131) -> (235, 131)
  line L3 (235, 131) -> (235, 50)
  dimension "d472" = 235
  dimension "d473" = 50
  dimension "d474" = 8
  dimension "d475" = 81
  constraint horizontal L0
  constraint vertical L1
  constraint horizontal L2
  constraint vertical L3
  measures "d472" horizontal distance of origin L0.start
  measures "d473" vertical distance of origin L0.start
  measures "d474" horizontal distance of L0.start L0.end
  measures "d475" vertical distance of L0.end L1.end
extrude "R04 low integral runner 0''" add sketch "草图7 (5)" along normal blind 10 bodies 5 in component "L2_Integrated"
ref_plane "工作平面8" through (0, 0, 0) normal (0, 0, 1) x (1, 0, 0) in component "L2_Integrated"
sketch "草图8 (5)" plane through (0, 0, 0) normal (0, 0, 1) x (1, 0, 0) in component "L2_Integrated"
  line L0 (419, 50) -> (427, 50)
  line L1 (427, 50) -> (427, 131)
  line L2 (427, 131) -> (419, 131)
  line L3 (419, 131) -> (419, 50)
  dimension "d480" = 419
  dimension "d481" = 50
  dimension "d482" = 8
  dimension "d483" = 81
  constraint horizontal L0
  constraint vertical L1
  constraint horizontal L2
  constraint vertical L3
  measures "d480" horizontal distance of origin L0.start
  measures "d481" vertical distance of origin L0.start
  measures "d482" horizontal distance of L0.start L0.end
  measures "d483" vertical distance of L0.end L1.end
extrude "R04 low integral runner 1''" add sketch "草图8 (5)" along normal blind 10 bodies 5 in component "L2_Integrated"
chamfer "R03 touch edge chamfer''''" distance 0.4 angle 45 5 edges at (331, 53, 30) (235, 96.5, 30) (427, 96.5, 30) (232, 95, 30) (430, 95, 30) on bodies 5 in component "L2_Integrated"
ref_plane "工作平面1" through (0, 0, 26) normal (0, 0, 1) x (1, 0, 0) in component "L2_RemovableGrate"
sketch "草图1 (6)" plane through (0, 0, 26) normal (0, 0, 1) x (1, 0, 0) in component "L2_RemovableGrate"
  line L0 (235.3, 53.3) -> (426.7, 53.3)
  line L1 (426.7, 53.3) -> (426.7, 136.7)
  line L2 (426.7, 136.7) -> (235.3, 136.7)
  line L3 (235.3, 136.7) -> (235.3, 53.3)
  dimension "d491" = 191.4
  dimension "d492" = 83.4
  constraint horizontal L0
  constraint vertical L1
  constraint horizontal L2
  constraint vertical L3
  measures "d491" horizontal distance of L0.start L0.end
  measures "d492" vertical distance of L0.end L1.end
extrude "Horizontal removable deck''" add sketch "草图1 (6)" along normal blind 4 separate body makes body 6 in component "L2_RemovableGrate"
ref_plane "工作平面2" through (0, 0, 26) normal (0, 0, 1) x (1, 0, 0) in component "L2_RemovableGrate"
sketch "草图2 (6)" plane through (0, 0, 26) normal (0, 0, 1) x (1, 0, 0) in component "L2_RemovableGrate"
  line L0 (249, 60.3) -> (253, 60.3)
  line L1 (253, 60.3) -> (253, 129.7)
  line L2 (253, 129.7) -> (249, 129.7)
  line L3 (249, 129.7) -> (249, 60.3)
  dimension "d497" = 249
  dimension "d499" = 4
  dimension "d500" = 69.4
  constraint horizontal L0
  constraint vertical L1
  constraint horizontal L2
  constraint vertical L3
  measures "d497" horizontal distance of origin L0.start
  measures "d499" horizontal distance of L0.start L0.end
  measures "d500" vertical distance of L0.end L1.end
extrude "Drain slot 1''" cut sketch "草图2 (6)" along normal blind 4 bodies 6 in component "L2_RemovableGrate"
ref_plane "工作平面3" through (0, 0, 26) normal (0, 0, 1) x (1, 0, 0) in component "L2_RemovableGrate"
sketch "草图3 (6)" plane through (0, 0, 26) normal (0, 0, 1) x (1, 0, 0) in component "L2_RemovableGrate"
  line L0 (259, 60.3) -> (263, 60.3)
  line L1 (263, 60.3) -> (263, 129.7)
  line L2 (263, 129.7) -> (259, 129.7)
  line L3 (259, 129.7) -> (259, 60.3)
  dimension "d505" = 259
  dimension "d507" = 4
  dimension "d508" = 69.4
  constraint horizontal L0
  constraint vertical L1
  constraint horizontal L2
  constraint vertical L3
  measures "d505" horizontal distance of origin L0.start
  measures "d507" horizontal distance of L0.start L0.end
  measures "d508" vertical distance of L0.end L1.end
extrude "Drain slot 2''" cut sketch "草图3 (6)" along normal blind 4 bodies 6 in component "L2_RemovableGrate"
ref_plane "工作平面4" through (0, 0, 26) normal (0, 0, 1) x (1, 0, 0) in component "L2_RemovableGrate"
sketch "草图4 (6)" plane through (0, 0, 26) normal (0, 0, 1) x (1, 0, 0) in component "L2_RemovableGrate"
  line L0 (269, 60.3) -> (273, 60.3)
  line L1 (273, 60.3) -> (273, 129.7)
  line L2 (273, 129.7) -> (269, 129.7)
  line L3 (269, 129.7) -> (269, 60.3)
  dimension "d513" = 269
  dimension "d515" = 4
  dimension "d516" = 69.4
  constraint horizontal L0
  constraint vertical L1
  constraint horizontal L2
  constraint vertical L3
  measures "d513" horizontal distance of origin L0.start
  measures "d515" horizontal distance of L0.start L0.end
  measures "d516" vertical distance of L0.end L1.end
extrude "Drain slot 3''" cut sketch "草图4 (6)" along normal blind 4 bodies 6 in component "L2_RemovableGrate"
ref_plane "工作平面5" through (0, 0, 26) normal (0, 0, 1) x (1, 0, 0) in component "L2_RemovableGrate"
sketch "草图5 (6)" plane through (0, 0, 26) normal (0, 0, 1) x (1, 0, 0) in component "L2_RemovableGrate"
  line L0 (279, 60.3) -> (283, 60.3)
  line L1 (283, 60.3) -> (283, 129.7)
  line L2 (283, 129.7) -> (279, 129.7)
  line L3 (279, 129.7) -> (279, 60.3)
  dimension "d521" = 279
  dimension "d523" = 4
  dimension "d524" = 69.4
  constraint horizontal L0
  constraint vertical L1
  constraint horizontal L2
  constraint vertical L3
  measures "d521" horizontal distance of origin L0.start
  measures "d523" horizontal distance of L0.start L0.end
  measures "d524" vertical distance of L0.end L1.end
extrude "Drain slot 4''" cut sketch "草图5 (6)" along normal blind 4 bodies 6 in component "L2_RemovableGrate"
ref_plane "工作平面6" through (0, 0, 26) normal (0, 0, 1) x (1, 0, 0) in component "L2_RemovableGrate"
sketch "草图6 (6)" plane through (0, 0, 26) normal (0, 0, 1) x (1, 0, 0) in component "L2_RemovableGrate"
  line L0 (289, 60.3) -> (293, 60.3)
  line L1 (293, 60.3) -> (293, 129.7)
  line L2 (293, 129.7) -> (289, 129.7)
  line L3 (289, 129.7) -> (289, 60.3)
  dimension "d529" = 289
  dimension "d531" = 4
  dimension "d532" = 69.4
  constraint horizontal L0
  constraint vertical L1
  constraint horizontal L2
  constraint vertical L3
  measures "d529" horizontal distance of origin L0.start
  measures "d531" horizontal distance of L0.start L0.end
  measures "d532" vertical distance of L0.end L1.end
extrude "Drain slot 5''" cut sketch "草图6 (6)" along normal blind 4 bodies 6 in component "L2_RemovableGrate"